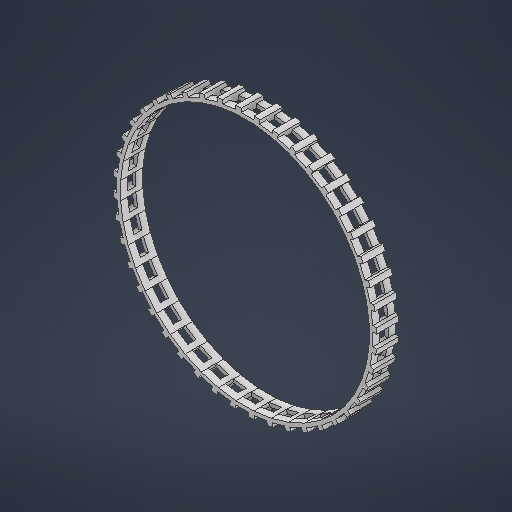
# Autodesk Inventor part: good_track
Saved by Autodesk Inventor 2026.2 (Build 302298010, 298A)
## iProperties
Created: 2026-07-08
Part Number: good_track
Material: Generic
Document SubType Name: Modeling
Designer: vicke
Density: 1 g/cm^3
Appearance: Default
Author: vicke
Autodesk Inventor part; units mm, degrees
ref_plane "YZ Plane" through (0, 0, 0) normal (1, 0, 0) x (0, 1, 0)
ref_plane "XZ Plane" through (0, 0, 0) normal (0, 1, 0) x (-1, 0, 0)
ref_plane "XY Plane" through (0, 0, 0) normal (0, 0, 1) x (1, 0, 0)
sketch "Sketch1" plane through (0, 0, 0) normal (0, 0, 1) x (1, 0, 0)
  line L0 (-5, 67) -> (5, 67)
  line L1 (0, 67) -> (-5, 67)
  line L2 (-5, 67) -> (-5, 71)
  line L3 (0, 67) -> (5, 67)
  line L4 (-5, 71) -> (-2, 71)
  line L5 (-2, 71) -> (-2, 67)
  line L6 (-2, 67) -> (-5, 67)
  line L7 (-5, 67) -> (-5, 71)
  line L8 (5, 67) -> (-2, 67)
  line L9 (-2, 67) -> (-2, 69)
  line L10 (-2, 69) -> (5, 69)
  line L11 (5, 69) -> (5, 67)
  line L12 (-14.4842, 65.6065) -> (-4.586, 67.0296)
  line L13 (-9.5351, 66.318) -> (-14.4842, 65.6065)
  line L14 (-9.5351, 66.318) -> (-4.586, 67.0296)
  line L15 (-11.5147, 66.0334) -> (-14.4842, 65.6065)
  line L16 (-4.586, 67.0296) -> (-11.5147, 66.0334)
  line L17 (-11.5147, 66.0334) -> (-11.7994, 68.013)
  line L18 (-11.7994, 68.013) -> (-4.8706, 69.0093)
  line L19 (-4.8706, 69.0093) -> (-4.586, 67.0296)
  line L20 (-14.4842, 65.6065) -> (-15.0535, 69.5657)
  line L21 (-15.0535, 69.5657) -> (-12.084, 69.9927)
  line L22 (-12.084, 69.9927) -> (-11.5147, 66.0334)
  line L23 (-14.4842, 65.6065) -> (-15.0535, 69.5657)
  line L24 (-23.6735, 62.8774) -> (-14.0786, 65.6947)
  line L25 (-18.8761, 64.286) -> (-23.6735, 62.8774)
  line L26 (-18.8761, 64.286) -> (-14.0786, 65.6947)
  line L27 (-20.7951, 63.7226) -> (-23.6735, 62.8774)
  line L28 (-14.0786, 65.6947) -> (-20.7951, 63.7226)
  line L29 (-20.7951, 63.7226) -> (-21.3585, 65.6416)
  line L30 (-21.3585, 65.6416) -> (-14.6421, 67.6137)
  line L31 (-14.6421, 67.6137) -> (-14.0786, 65.6947)
  line L32 (-23.6735, 62.8774) -> (-24.8005, 66.7153)
  line L33 (-24.8005, 66.7153) -> (-21.922, 67.5605)
  line L34 (-21.922, 67.5605) -> (-20.7951, 63.7226)
  line L35 (-23.6735, 62.8774) -> (-24.8005, 66.7153)
  line L36 (-32.381, 58.8683) -> (-23.2846, 63.0224)
  line L37 (-27.8328, 60.9453) -> (-32.381, 58.8683)
  line L38 (-27.8328, 60.9453) -> (-23.2846, 63.0224)
  line L39 (-29.6521, 60.1145) -> (-32.381, 58.8683)
  line L40 (-23.2846, 63.0224) -> (-29.6521, 60.1145)
  line L41 (-29.6521, 60.1145) -> (-30.4829, 61.9338)
  line L42 (-30.4829, 61.9338) -> (-24.1155, 64.8417)
  line L43 (-24.1155, 64.8417) -> (-23.2846, 63.0224)
  line L44 (-32.381, 58.8683) -> (-34.0426, 62.5068)
  line L45 (-34.0426, 62.5068) -> (-31.3137, 63.753)
  line L46 (-31.3137, 63.753) -> (-29.6521, 60.1145)
  line L47 (-32.381, 58.8683) -> (-34.0426, 62.5068)
  line L48 (-40.4292, 53.6608) -> (-32.0167, 59.0672)
  line L49 (-36.2229, 56.364) -> (-40.4292, 53.6608)
  line L50 (-36.2229, 56.364) -> (-32.0167, 59.0672)
  line L51 (-37.9054, 55.2827) -> (-40.4292, 53.6608)
  line L52 (-32.0167, 59.0672) -> (-37.9054, 55.2827)
  line L53 (-37.9054, 55.2827) -> (-38.9867, 56.9652)
  line L54 (-38.9867, 56.9652) -> (-33.0979, 60.7497)
  line L55 (-33.0979, 60.7497) -> (-32.0167, 59.0672)
  line L56 (-40.4292, 53.6608) -> (-42.5918, 57.0258)
  line L57 (-42.5918, 57.0258) -> (-40.068, 58.6477)
  line L58 (-40.068, 58.6477) -> (-37.9054, 55.2827)
  line L59 (-40.4292, 53.6608) -> (-42.5918, 57.0258)
  line L60 (-47.6544, 47.3609) -> (-40.0969, 53.9095)
  line L61 (-43.8757, 50.6352) -> (-47.6544, 47.3609)
  line L62 (-43.8757, 50.6352) -> (-40.0969, 53.9095)
  line L63 (-45.3872, 49.3255) -> (-47.6544, 47.3609)
  line L64 (-40.0969, 53.9095) -> (-45.3872, 49.3255)
  line L65 (-45.3872, 49.3255) -> (-46.6969, 50.837)
  line L66 (-46.6969, 50.837) -> (-41.4066, 55.421)
  line L67 (-41.4066, 55.421) -> (-40.0969, 53.9095)
  line L68 (-47.6544, 47.3609) -> (-50.2739, 50.3839)
  line L69 (-50.2739, 50.3839) -> (-48.0066, 52.3485)
  line L70 (-48.0066, 52.3485) -> (-45.3872, 49.3255)
  line L71 (-47.6544, 47.3609) -> (-50.2739, 50.3839)
  line L72 (-53.9095, 40.0969) -> (-47.3609, 47.6544)
  line L73 (-50.6352, 43.8757) -> (-53.9095, 40.0969)
  line L74 (-50.6352, 43.8757) -> (-47.3609, 47.6544)
  line L75 (-51.9449, 42.3642) -> (-53.9095, 40.0969)
  line L76 (-47.3609, 47.6544) -> (-51.9449, 42.3642)
  line L77 (-51.9449, 42.3642) -> (-53.4564, 43.6739)
  line L78 (-53.4564, 43.6739) -> (-48.8724, 48.9641)
  line L79 (-48.8724, 48.9641) -> (-47.3609, 47.6544)
  line L80 (-53.9095, 40.0969) -> (-56.9325, 42.7164)
  line L81 (-56.9325, 42.7164) -> (-54.9679, 44.9836)
  line L82 (-54.9679, 44.9836) -> (-51.9449, 42.3642)
  line L83 (-53.9095, 40.0969) -> (-56.9325, 42.7164)
  line L84 (-59.0672, 32.0167) -> (-53.6608, 40.4292)
  line L85 (-56.364, 36.2229) -> (-59.0672, 32.0167)
  line L86 (-56.364, 36.2229) -> (-53.6608, 40.4292)
  line L87 (-57.4453, 34.5404) -> (-59.0672, 32.0167)
  line L88 (-53.6608, 40.4292) -> (-57.4453, 34.5404)
  line L89 (-57.4453, 34.5404) -> (-59.1278, 35.6217)
  line L90 (-59.1278, 35.6217) -> (-55.3433, 41.5105)
  line L91 (-55.3433, 41.5105) -> (-53.6608, 40.4292)
  line L92 (-59.0672, 32.0167) -> (-62.4322, 34.1792)
  line L93 (-62.4322, 34.1792) -> (-60.8103, 36.703)
  line L94 (-60.8103, 36.703) -> (-57.4453, 34.5404)
  line L95 (-59.0672, 32.0167) -> (-62.4322, 34.1792)
  line L96 (-63.0224, 23.2846) -> (-58.8683, 32.381)
  line L97 (-60.9453, 27.8328) -> (-63.0224, 23.2846)
  line L98 (-60.9453, 27.8328) -> (-58.8683, 32.381)
  line L99 (-61.7762, 26.0135) -> (-63.0224, 23.2846)
  line L100 (-58.8683, 32.381) -> (-61.7762, 26.0135)
  line L101 (-61.7762, 26.0135) -> (-63.5954, 26.8444)
  line L102 (-63.5954, 26.8444) -> (-60.6875, 33.2118)
  line L103 (-60.6875, 33.2118) -> (-58.8683, 32.381)
  line L104 (-63.0224, 23.2846) -> (-66.6609, 24.9463)
  line L105 (-66.6609, 24.9463) -> (-65.4147, 27.6752)
  line L106 (-65.4147, 27.6752) -> (-61.7762, 26.0135)
  line L107 (-63.0224, 23.2846) -> (-66.6609, 24.9463)
  line L108 (-65.6947, 14.0786) -> (-62.8774, 23.6735)
  line L109 (-64.286, 18.8761) -> (-65.6947, 14.0786)
  line L110 (-64.286, 18.8761) -> (-62.8774, 23.6735)
  line L111 (-64.8495, 16.9571) -> (-65.6947, 14.0786)
  line L112 (-62.8774, 23.6735) -> (-64.8495, 16.9571)
  line L113 (-64.8495, 16.9571) -> (-66.7685, 17.5206)
  line L114 (-66.7685, 17.5206) -> (-64.7964, 24.237)
  line L115 (-64.7964, 24.237) -> (-62.8774, 23.6735)
  line L116 (-65.6947, 14.0786) -> (-69.5327, 15.2055)
  line L117 (-69.5327, 15.2055) -> (-68.6875, 18.084)
  line L118 (-68.6875, 18.084) -> (-64.8495, 16.9571)
  line L119 (-65.6947, 14.0786) -> (-69.5327, 15.2055)
  line L120 (-67.0296, 4.586) -> (-65.6065, 14.4842)
  line L121 (-66.318, 9.5351) -> (-67.0296, 4.586)
  line L122 (-66.318, 9.5351) -> (-65.6065, 14.4842)
  line L123 (-66.6027, 7.5555) -> (-67.0296, 4.586)
  line L124 (-65.6065, 14.4842) -> (-66.6027, 7.5555)
  line L125 (-66.6027, 7.5555) -> (-68.5823, 7.8401)
  line L126 (-68.5823, 7.8401) -> (-67.5861, 14.7688)
  line L127 (-67.5861, 14.7688) -> (-65.6065, 14.4842)
  line L128 (-67.0296, 4.586) -> (-70.9889, 5.1552)
  line L129 (-70.9889, 5.1552) -> (-70.562, 8.1247)
  line L130 (-70.562, 8.1247) -> (-66.6027, 7.5555)
  line L131 (-67.0296, 4.586) -> (-70.9889, 5.1552)
  line L132 (-67, -5) -> (-67, 5)
  line L133 (-67, 0) -> (-67, -5)
  line L134 (-67, 0) -> (-67, 5)
  line L135 (-67, -2) -> (-67, -5)
  line L136 (-67, 5) -> (-67, -2)
  line L137 (-67, -2) -> (-69, -2)
  line L138 (-69, -2) -> (-69, 5)
  line L139 (-69, 5) -> (-67, 5)
  line L140 (-67, -5) -> (-71, -5)
  line L141 (-71, -5) -> (-71, -2)
  line L142 (-71, -2) -> (-67, -2)
  line L143 (-67, -5) -> (-71, -5)
  line L144 (-65.6065, -14.4842) -> (-67.0296, -4.586)
  line L145 (-66.318, -9.5351) -> (-65.6065, -14.4842)
  line L146 (-66.318, -9.5351) -> (-67.0296, -4.586)
  line L147 (-66.0334, -11.5147) -> (-65.6065, -14.4842)
  line L148 (-67.0296, -4.586) -> (-66.0334, -11.5147)
  line L149 (-66.0334, -11.5147) -> (-68.013, -11.7994)
  line L150 (-68.013, -11.7994) -> (-69.0093, -4.8706)
  line L151 (-69.0093, -4.8706) -> (-67.0296, -4.586)
  line L152 (-65.6065, -14.4842) -> (-69.5657, -15.0535)
  line L153 (-69.5657, -15.0535) -> (-69.9927, -12.084)
  line L154 (-69.9927, -12.084) -> (-66.0334, -11.5147)
  line L155 (-65.6065, -14.4842) -> (-69.5657, -15.0535)
  line L156 (-62.8774, -23.6735) -> (-65.6947, -14.0786)
  line L157 (-64.286, -18.8761) -> (-62.8774, -23.6735)
  line L158 (-64.286, -18.8761) -> (-65.6947, -14.0786)
  line L159 (-63.7226, -20.7951) -> (-62.8774, -23.6735)
  line L160 (-65.6947, -14.0786) -> (-63.7226, -20.7951)
  line L161 (-63.7226, -20.7951) -> (-65.6416, -21.3585)
  line L162 (-65.6416, -21.3585) -> (-67.6137, -14.6421)
  line L163 (-67.6137, -14.6421) -> (-65.6947, -14.0786)
  line L164 (-62.8774, -23.6735) -> (-66.7153, -24.8005)
  line L165 (-66.7153, -24.8005) -> (-67.5605, -21.922)
  line L166 (-67.5605, -21.922) -> (-63.7226, -20.7951)
  line L167 (-62.8774, -23.6735) -> (-66.7153, -24.8005)
  line L168 (-58.8683, -32.381) -> (-63.0224, -23.2846)
  line L169 (-60.9453, -27.8328) -> (-58.8683, -32.381)
  line L170 (-60.9453, -27.8328) -> (-63.0224, -23.2846)
  line L171 (-60.1145, -29.6521) -> (-58.8683, -32.381)
  line L172 (-63.0224, -23.2846) -> (-60.1145, -29.6521)
  line L173 (-60.1145, -29.6521) -> (-61.9338, -30.4829)
  line L174 (-61.9338, -30.4829) -> (-64.8417, -24.1155)
  line L175 (-64.8417, -24.1155) -> (-63.0224, -23.2846)
  line L176 (-58.8683, -32.381) -> (-62.5068, -34.0426)
  line L177 (-62.5068, -34.0426) -> (-63.753, -31.3137)
  line L178 (-63.753, -31.3137) -> (-60.1145, -29.6521)
  line L179 (-58.8683, -32.381) -> (-62.5068, -34.0426)
  line L180 (-53.6608, -40.4292) -> (-59.0672, -32.0167)
  line L181 (-56.364, -36.2229) -> (-53.6608, -40.4292)
  line L182 (-56.364, -36.2229) -> (-59.0672, -32.0167)
  line L183 (-55.2827, -37.9054) -> (-53.6608, -40.4292)
  line L184 (-59.0672, -32.0167) -> (-55.2827, -37.9054)
  line L185 (-55.2827, -37.9054) -> (-56.9652, -38.9867)
  line L186 (-56.9652, -38.9867) -> (-60.7497, -33.0979)
  line L187 (-60.7497, -33.0979) -> (-59.0672, -32.0167)
  line L188 (-53.6608, -40.4292) -> (-57.0258, -42.5918)
  line L189 (-57.0258, -42.5918) -> (-58.6477, -40.068)
  line L190 (-58.6477, -40.068) -> (-55.2827, -37.9054)
  line L191 (-53.6608, -40.4292) -> (-57.0258, -42.5918)
  line L192 (-47.3609, -47.6544) -> (-53.9095, -40.0969)
  line L193 (-50.6352, -43.8757) -> (-47.3609, -47.6544)
  line L194 (-50.6352, -43.8757) -> (-53.9095, -40.0969)
  line L195 (-49.3255, -45.3872) -> (-47.3609, -47.6544)
  line L196 (-53.9095, -40.0969) -> (-49.3255, -45.3872)
  line L197 (-49.3255, -45.3872) -> (-50.837, -46.6969)
  line L198 (-50.837, -46.6969) -> (-55.421, -41.4066)
  line L199 (-55.421, -41.4066) -> (-53.9095, -40.0969)
  line L200 (-47.3609, -47.6544) -> (-50.3839, -50.2739)
  line L201 (-50.3839, -50.2739) -> (-52.3485, -48.0066)
  line L202 (-52.3485, -48.0066) -> (-49.3255, -45.3872)
  line L203 (-47.3609, -47.6544) -> (-50.3839, -50.2739)
  line L204 (-40.0969, -53.9095) -> (-47.6544, -47.3609)
  line L205 (-43.8757, -50.6352) -> (-40.0969, -53.9095)
  line L206 (-43.8757, -50.6352) -> (-47.6544, -47.3609)
  line L207 (-42.3642, -51.9449) -> (-40.0969, -53.9095)
  line L208 (-47.6544, -47.3609) -> (-42.3642, -51.9449)
  line L209 (-42.3642, -51.9449) -> (-43.6739, -53.4564)
  line L210 (-43.6739, -53.4564) -> (-48.9641, -48.8724)
  line L211 (-48.9641, -48.8724) -> (-47.6544, -47.3609)
  line L212 (-40.0969, -53.9095) -> (-42.7164, -56.9325)
  line L213 (-42.7164, -56.9325) -> (-44.9836, -54.9679)
  line L214 (-44.9836, -54.9679) -> (-42.3642, -51.9449)
  line L215 (-40.0969, -53.9095) -> (-42.7164, -56.9325)
  line L216 (-32.0167, -59.0672) -> (-40.4292, -53.6608)
  line L217 (-36.2229, -56.364) -> (-32.0167, -59.0672)
  line L218 (-36.2229, -56.364) -> (-40.4292, -53.6608)
  line L219 (-34.5404, -57.4453) -> (-32.0167, -59.0672)
  line L220 (-40.4292, -53.6608) -> (-34.5404, -57.4453)
  line L221 (-34.5404, -57.4453) -> (-35.6217, -59.1278)
  line L222 (-35.6217, -59.1278) -> (-41.5105, -55.3433)
  line L223 (-41.5105, -55.3433) -> (-40.4292, -53.6608)
  line L224 (-32.0167, -59.0672) -> (-34.1792, -62.4322)
  line L225 (-34.1792, -62.4322) -> (-36.703, -60.8103)
  line L226 (-36.703, -60.8103) -> (-34.5404, -57.4453)
  line L227 (-32.0167, -59.0672) -> (-34.1792, -62.4322)
  line L228 (-23.2846, -63.0224) -> (-32.381, -58.8683)
  line L229 (-27.8328, -60.9453) -> (-23.2846, -63.0224)
  line L230 (-27.8328, -60.9453) -> (-32.381, -58.8683)
  line L231 (-26.0135, -61.7762) -> (-23.2846, -63.0224)
  line L232 (-32.381, -58.8683) -> (-26.0135, -61.7762)
  line L233 (-26.0135, -61.7762) -> (-26.8444, -63.5954)
  line L234 (-26.8444, -63.5954) -> (-33.2118, -60.6875)
  line L235 (-33.2118, -60.6875) -> (-32.381, -58.8683)
  line L236 (-23.2846, -63.0224) -> (-24.9463, -66.6609)
  line L237 (-24.9463, -66.6609) -> (-27.6752, -65.4147)
  line L238 (-27.6752, -65.4147) -> (-26.0135, -61.7762)
  line L239 (-23.2846, -63.0224) -> (-24.9463, -66.6609)
  line L240 (-14.0786, -65.6947) -> (-23.6735, -62.8774)
  line L241 (-18.8761, -64.286) -> (-14.0786, -65.6947)
  line L242 (-18.8761, -64.286) -> (-23.6735, -62.8774)
  line L243 (-16.9571, -64.8495) -> (-14.0786, -65.6947)
  line L244 (-23.6735, -62.8774) -> (-16.9571, -64.8495)
  line L245 (-16.9571, -64.8495) -> (-17.5206, -66.7685)
  line L246 (-17.5206, -66.7685) -> (-24.237, -64.7964)
  line L247 (-24.237, -64.7964) -> (-23.6735, -62.8774)
  line L248 (-14.0786, -65.6947) -> (-15.2055, -69.5327)
  line L249 (-15.2055, -69.5327) -> (-18.084, -68.6875)
  line L250 (-18.084, -68.6875) -> (-16.9571, -64.8495)
  line L251 (-14.0786, -65.6947) -> (-15.2055, -69.5327)
  line L252 (-4.586, -67.0296) -> (-14.4842, -65.6065)
  line L253 (-9.5351, -66.318) -> (-4.586, -67.0296)
  line L254 (-9.5351, -66.318) -> (-14.4842, -65.6065)
  line L255 (-7.5555, -66.6027) -> (-4.586, -67.0296)
  line L256 (-14.4842, -65.6065) -> (-7.5555, -66.6027)
  line L257 (-7.5555, -66.6027) -> (-7.8401, -68.5823)
  line L258 (-7.8401, -68.5823) -> (-14.7688, -67.5861)
  line L259 (-14.7688, -67.5861) -> (-14.4842, -65.6065)
  line L260 (-4.586, -67.0296) -> (-5.1552, -70.9889)
  line L261 (-5.1552, -70.9889) -> (-8.1247, -70.562)
  line L262 (-8.1247, -70.562) -> (-7.5555, -66.6027)
  line L263 (-4.586, -67.0296) -> (-5.1552, -70.9889)
  line L264 (5, -67) -> (-5, -67)
  line L265 (0, -67) -> (5, -67)
  line L266 (0, -67) -> (-5, -67)
  line L267 (2, -67) -> (5, -67)
  line L268 (-5, -67) -> (2, -67)
  line L269 (2, -67) -> (2, -69)
  line L270 (2, -69) -> (-5, -69)
  line L271 (-5, -69) -> (-5, -67)
  line L272 (5, -67) -> (5, -71)
  line L273 (5, -71) -> (2, -71)
  line L274 (2, -71) -> (2, -67)
  line L275 (5, -67) -> (5, -71)
  line L276 (14.4842, -65.6065) -> (4.586, -67.0296)
  line L277 (9.5351, -66.318) -> (14.4842, -65.6065)
  line L278 (9.5351, -66.318) -> (4.586, -67.0296)
  line L279 (11.5147, -66.0334) -> (14.4842, -65.6065)
  line L280 (4.586, -67.0296) -> (11.5147, -66.0334)
  line L281 (11.5147, -66.0334) -> (11.7994, -68.013)
  line L282 (11.7994, -68.013) -> (4.8706, -69.0093)
  line L283 (4.8706, -69.0093) -> (4.586, -67.0296)
  line L284 (14.4842, -65.6065) -> (15.0535, -69.5657)
  line L285 (15.0535, -69.5657) -> (12.084, -69.9927)
  line L286 (12.084, -69.9927) -> (11.5147, -66.0334)
  line L287 (14.4842, -65.6065) -> (15.0535, -69.5657)
  line L288 (23.6735, -62.8774) -> (14.0786, -65.6947)
  line L289 (18.8761, -64.286) -> (23.6735, -62.8774)
  line L290 (18.8761, -64.286) -> (14.0786, -65.6947)
  line L291 (20.7951, -63.7226) -> (23.6735, -62.8774)
  line L292 (14.0786, -65.6947) -> (20.7951, -63.7226)
  line L293 (20.7951, -63.7226) -> (21.3585, -65.6416)
  line L294 (21.3585, -65.6416) -> (14.6421, -67.6137)
  line L295 (14.6421, -67.6137) -> (14.0786, -65.6947)
  line L296 (23.6735, -62.8774) -> (24.8005, -66.7153)
  line L297 (24.8005, -66.7153) -> (21.922, -67.5605)
  line L298 (21.922, -67.5605) -> (20.7951, -63.7226)
  line L299 (23.6735, -62.8774) -> (24.8005, -66.7153)
  line L300 (32.381, -58.8683) -> (23.2846, -63.0224)
  line L301 (27.8328, -60.9453) -> (32.381, -58.8683)
  line L302 (27.8328, -60.9453) -> (23.2846, -63.0224)
  line L303 (29.6521, -60.1145) -> (32.381, -58.8683)
  line L304 (23.2846, -63.0224) -> (29.6521, -60.1145)
  line L305 (29.6521, -60.1145) -> (30.4829, -61.9338)
  line L306 (30.4829, -61.9338) -> (24.1155, -64.8417)
  line L307 (24.1155, -64.8417) -> (23.2846, -63.0224)
  line L308 (32.381, -58.8683) -> (34.0426, -62.5068)
  line L309 (34.0426, -62.5068) -> (31.3137, -63.753)
  line L310 (31.3137, -63.753) -> (29.6521, -60.1145)
  line L311 (32.381, -58.8683) -> (34.0426, -62.5068)
  line L312 (40.4292, -53.6608) -> (32.0167, -59.0672)
  line L313 (36.2229, -56.364) -> (40.4292, -53.6608)
  line L314 (36.2229, -56.364) -> (32.0167, -59.0672)
  line L315 (37.9054, -55.2827) -> (40.4292, -53.6608)
  line L316 (32.0167, -59.0672) -> (37.9054, -55.2827)
  line L317 (37.9054, -55.2827) -> (38.9867, -56.9652)
  line L318 (38.9867, -56.9652) -> (33.0979, -60.7497)
  line L319 (33.0979, -60.7497) -> (32.0167, -59.0672)
  line L320 (40.4292, -53.6608) -> (42.5918, -57.0258)
  line L321 (42.5918, -57.0258) -> (40.068, -58.6477)
  line L322 (40.068, -58.6477) -> (37.9054, -55.2827)
  line L323 (40.4292, -53.6608) -> (42.5918, -57.0258)
  line L324 (47.6544, -47.3609) -> (40.0969, -53.9095)
  line L325 (43.8757, -50.6352) -> (47.6544, -47.3609)
  line L326 (43.8757, -50.6352) -> (40.0969, -53.9095)
  line L327 (45.3872, -49.3255) -> (47.6544, -47.3609)
  line L328 (40.0969, -53.9095) -> (45.3872, -49.3255)
  line L329 (45.3872, -49.3255) -> (46.6969, -50.837)
  line L330 (46.6969, -50.837) -> (41.4066, -55.421)
  line L331 (41.4066, -55.421) -> (40.0969, -53.9095)
  line L332 (47.6544, -47.3609) -> (50.2739, -50.3839)
  line L333 (50.2739, -50.3839) -> (48.0066, -52.3485)
  line L334 (48.0066, -52.3485) -> (45.3872, -49.3255)
  line L335 (47.6544, -47.3609) -> (50.2739, -50.3839)
  line L336 (53.9095, -40.0969) -> (47.3609, -47.6544)
  line L337 (50.6352, -43.8757) -> (53.9095, -40.0969)
  line L338 (50.6352, -43.8757) -> (47.3609, -47.6544)
  line L339 (51.9449, -42.3642) -> (53.9095, -40.0969)
  line L340 (47.3609, -47.6544) -> (51.9449, -42.3642)
  line L341 (51.9449, -42.3642) -> (53.4564, -43.6739)
  line L342 (53.4564, -43.6739) -> (48.8724, -48.9641)
  line L343 (48.8724, -48.9641) -> (47.3609, -47.6544)
  line L344 (53.9095, -40.0969) -> (56.9325, -42.7164)
  line L345 (56.9325, -42.7164) -> (54.9679, -44.9836)
  line L346 (54.9679, -44.9836) -> (51.9449, -42.3642)
  line L347 (53.9095, -40.0969) -> (56.9325, -42.7164)
  line L348 (59.0672, -32.0167) -> (53.6608, -40.4292)
  line L349 (56.364, -36.2229) -> (59.0672, -32.0167)
  line L350 (56.364, -36.2229) -> (53.6608, -40.4292)
  line L351 (57.4453, -34.5404) -> (59.0672, -32.0167)
  line L352 (53.6608, -40.4292) -> (57.4453, -34.5404)
  line L353 (57.4453, -34.5404) -> (59.1278, -35.6217)
  line L354 (59.1278, -35.6217) -> (55.3433, -41.5105)
  line L355 (55.3433, -41.5105) -> (53.6608, -40.4292)
  line L356 (59.0672, -32.0167) -> (62.4322, -34.1792)
  line L357 (62.4322, -34.1792) -> (60.8103, -36.703)
  line L358 (60.8103, -36.703) -> (57.4453, -34.5404)
  line L359 (59.0672, -32.0167) -> (62.4322, -34.1792)
  line L360 (63.0224, -23.2846) -> (58.8683, -32.381)
  line L361 (60.9453, -27.8328) -> (63.0224, -23.2846)
  line L362 (60.9453, -27.8328) -> (58.8683, -32.381)
  line L363 (61.7762, -26.0135) -> (63.0224, -23.2846)
  line L364 (58.8683, -32.381) -> (61.7762, -26.0135)
  line L365 (61.7762, -26.0135) -> (63.5954, -26.8444)
  line L366 (63.5954, -26.8444) -> (60.6875, -33.2118)
  line L367 (60.6875, -33.2118) -> (58.8683, -32.381)
  line L368 (63.0224, -23.2846) -> (66.6609, -24.9463)
  line L369 (66.6609, -24.9463) -> (65.4147, -27.6752)
  line L370 (65.4147, -27.6752) -> (61.7762, -26.0135)
  line L371 (63.0224, -23.2846) -> (66.6609, -24.9463)
  line L372 (65.6947, -14.0786) -> (62.8774, -23.6735)
  line L373 (64.286, -18.8761) -> (65.6947, -14.0786)
  line L374 (64.286, -18.8761) -> (62.8774, -23.6735)
  line L375 (64.8495, -16.9571) -> (65.6947, -14.0786)
  line L376 (62.8774, -23.6735) -> (64.8495, -16.9571)
  line L377 (64.8495, -16.9571) -> (66.7685, -17.5206)
  line L378 (66.7685, -17.5206) -> (64.7964, -24.237)
  line L379 (64.7964, -24.237) -> (62.8774, -23.6735)
  line L380 (65.6947, -14.0786) -> (69.5327, -15.2055)
  line L381 (69.5327, -15.2055) -> (68.6875, -18.084)
  line L382 (68.6875, -18.084) -> (64.8495, -16.9571)
  line L383 (65.6947, -14.0786) -> (69.5327, -15.2055)
  line L384 (67.0296, -4.586) -> (65.6065, -14.4842)
  line L385 (66.318, -9.5351) -> (67.0296, -4.586)
  line L386 (66.318, -9.5351) -> (65.6065, -14.4842)
  line L387 (66.6027, -7.5555) -> (67.0296, -4.586)
  line L388 (65.6065, -14.4842) -> (66.6027, -7.5555)
  line L389 (66.6027, -7.5555) -> (68.5823, -7.8401)
  line L390 (68.5823, -7.8401) -> (67.5861, -14.7688)
  line L391 (67.5861, -14.7688) -> (65.6065, -14.4842)
  line L392 (67.0296, -4.586) -> (70.9889, -5.1552)
  line L393 (70.9889, -5.1552) -> (70.562, -8.1247)
  line L394 (70.562, -8.1247) -> (66.6027, -7.5555)
  line L395 (67.0296, -4.586) -> (70.9889, -5.1552)
  line L396 (67, 5) -> (67, -5)
  line L397 (67, 0) -> (67, 5)
  line L398 (67, 0) -> (67, -5)
  line L399 (67, 2) -> (67, 5)
  line L400 (67, -5) -> (67, 2)
  line L401 (67, 2) -> (69, 2)
  line L402 (69, 2) -> (69, -5)
  line L403 (69, -5) -> (67, -5)
  line L404 (67, 5) -> (71, 5)
  line L405 (71, 5) -> (71, 2)
  line L406 (71, 2) -> (67, 2)
  line L407 (67, 5) -> (71, 5)
  line L408 (65.6065, 14.4842) -> (67.0296, 4.586)
  line L409 (66.318, 9.5351) -> (65.6065, 14.4842)
  line L410 (66.318, 9.5351) -> (67.0296, 4.586)
  line L411 (66.0334, 11.5147) -> (65.6065, 14.4842)
  line L412 (67.0296, 4.586) -> (66.0334, 11.5147)
  line L413 (66.0334, 11.5147) -> (68.013, 11.7994)
  line L414 (68.013, 11.7994) -> (69.0093, 4.8706)
  line L415 (69.0093, 4.8706) -> (67.0296, 4.586)
  line L416 (65.6065, 14.4842) -> (69.5657, 15.0535)
  line L417 (69.5657, 15.0535) -> (69.9927, 12.084)
  line L418 (69.9927, 12.084) -> (66.0334, 11.5147)
  line L419 (65.6065, 14.4842) -> (69.5657, 15.0535)
  line L420 (62.8774, 23.6735) -> (65.6947, 14.0786)
  line L421 (64.286, 18.8761) -> (62.8774, 23.6735)
  line L422 (64.286, 18.8761) -> (65.6947, 14.0786)
  line L423 (63.7226, 20.7951) -> (62.8774, 23.6735)
  line L424 (65.6947, 14.0786) -> (63.7226, 20.7951)
  line L425 (63.7226, 20.7951) -> (65.6416, 21.3585)
  line L426 (65.6416, 21.3585) -> (67.6137, 14.6421)
  line L427 (67.6137, 14.6421) -> (65.6947, 14.0786)
  line L428 (62.8774, 23.6735) -> (66.7153, 24.8005)
  line L429 (66.7153, 24.8005) -> (67.5605, 21.922)
  line L430 (67.5605, 21.922) -> (63.7226, 20.7951)
  line L431 (62.8774, 23.6735) -> (66.7153, 24.8005)
  line L432 (58.8683, 32.381) -> (63.0224, 23.2846)
  line L433 (60.9453, 27.8328) -> (58.8683, 32.381)
  line L434 (60.9453, 27.8328) -> (63.0224, 23.2846)
  line L435 (60.1145, 29.6521) -> (58.8683, 32.381)
  line L436 (63.0224, 23.2846) -> (60.1145, 29.6521)
  line L437 (60.1145, 29.6521) -> (61.9338, 30.4829)
  line L438 (61.9338, 30.4829) -> (64.8417, 24.1155)
  line L439 (64.8417, 24.1155) -> (63.0224, 23.2846)
  line L440 (58.8683, 32.381) -> (62.5068, 34.0426)
  line L441 (62.5068, 34.0426) -> (63.753, 31.3137)
  line L442 (63.753, 31.3137) -> (60.1145, 29.6521)
  line L443 (58.8683, 32.381) -> (62.5068, 34.0426)
  line L444 (53.6608, 40.4292) -> (59.0672, 32.0167)
  line L445 (56.364, 36.2229) -> (53.6608, 40.4292)
  line L446 (56.364, 36.2229) -> (59.0672, 32.0167)
  line L447 (55.2827, 37.9054) -> (53.6608, 40.4292)
  line L448 (59.0672, 32.0167) -> (55.2827, 37.9054)
  line L449 (55.2827, 37.9054) -> (56.9652, 38.9867)
  line L450 (56.9652, 38.9867) -> (60.7497, 33.0979)
  line L451 (60.7497, 33.0979) -> (59.0672, 32.0167)
  line L452 (53.6608, 40.4292) -> (57.0258, 42.5918)
  line L453 (57.0258, 42.5918) -> (58.6477, 40.068)
  line L454 (58.6477, 40.068) -> (55.2827, 37.9054)
  line L455 (53.6608, 40.4292) -> (57.0258, 42.5918)
  line L456 (47.3609, 47.6544) -> (53.9095, 40.0969)
  line L457 (50.6352, 43.8757) -> (47.3609, 47.6544)
  line L458 (50.6352, 43.8757) -> (53.9095, 40.0969)
  line L459 (49.3255, 45.3872) -> (47.3609, 47.6544)
  line L460 (53.9095, 40.0969) -> (49.3255, 45.3872)
  line L461 (49.3255, 45.3872) -> (50.837, 46.6969)
  line L462 (50.837, 46.6969) -> (55.421, 41.4066)
  line L463 (55.421, 41.4066) -> (53.9095, 40.0969)
  line L464 (47.3609, 47.6544) -> (50.3839, 50.2739)
  line L465 (50.3839, 50.2739) -> (52.3485, 48.0066)
  line L466 (52.3485, 48.0066) -> (49.3255, 45.3872)
  line L467 (47.3609, 47.6544) -> (50.3839, 50.2739)
  line L468 (40.0969, 53.9095) -> (47.6544, 47.3609)
  line L469 (43.8757, 50.6352) -> (40.0969, 53.9095)
  line L470 (43.8757, 50.6352) -> (47.6544, 47.3609)
  line L471 (42.3642, 51.9449) -> (40.0969, 53.9095)
  line L472 (47.6544, 47.3609) -> (42.3642, 51.9449)
  line L473 (42.3642, 51.9449) -> (43.6739, 53.4564)
  line L474 (43.6739, 53.4564) -> (48.9641, 48.8724)
  line L475 (48.9641, 48.8724) -> (47.6544, 47.3609)
  line L476 (40.0969, 53.9095) -> (42.7164, 56.9325)
  line L477 (42.7164, 56.9325) -> (44.9836, 54.9679)
  line L478 (44.9836, 54.9679) -> (42.3642, 51.9449)
  line L479 (40.0969, 53.9095) -> (42.7164, 56.9325)
  line L480 (32.0167, 59.0672) -> (40.4292, 53.6608)
  line L481 (36.2229, 56.364) -> (32.0167, 59.0672)
  line L482 (36.2229, 56.364) -> (40.4292, 53.6608)
  line L483 (34.5404, 57.4453) -> (32.0167, 59.0672)
  line L484 (40.4292, 53.6608) -> (34.5404, 57.4453)
  line L485 (34.5404, 57.4453) -> (35.6217, 59.1278)
  line L486 (35.6217, 59.1278) -> (41.5105, 55.3433)
  line L487 (41.5105, 55.3433) -> (40.4292, 53.6608)
  line L488 (32.0167, 59.0672) -> (34.1792, 62.4322)
  line L489 (34.1792, 62.4322) -> (36.703, 60.8103)
  line L490 (36.703, 60.8103) -> (34.5404, 57.4453)
  line L491 (32.0167, 59.0672) -> (34.1792, 62.4322)
  line L492 (23.2846, 63.0224) -> (32.381, 58.8683)
  line L493 (27.8328, 60.9453) -> (23.2846, 63.0224)
  line L494 (27.8328, 60.9453) -> (32.381, 58.8683)
  line L495 (26.0135, 61.7762) -> (23.2846, 63.0224)
  line L496 (32.381, 58.8683) -> (26.0135, 61.7762)
  line L497 (26.0135, 61.7762) -> (26.8444, 63.5954)
  line L498 (26.8444, 63.5954) -> (33.2118, 60.6875)
  line L499 (33.2118, 60.6875) -> (32.381, 58.8683)
  line L500 (23.2846, 63.0224) -> (24.9463, 66.6609)
  line L501 (24.9463, 66.6609) -> (27.6752, 65.4147)
  line L502 (27.6752, 65.4147) -> (26.0135, 61.7762)
  line L503 (23.2846, 63.0224) -> (24.9463, 66.6609)
  line L504 (14.0786, 65.6947) -> (23.6735, 62.8774)
  line L505 (18.8761, 64.286) -> (14.0786, 65.6947)
  line L506 (18.8761, 64.286) -> (23.6735, 62.8774)
  line L507 (16.9571, 64.8495) -> (14.0786, 65.6947)
  line L508 (23.6735, 62.8774) -> (16.9571, 64.8495)
  line L509 (16.9571, 64.8495) -> (17.5206, 66.7685)
  line L510 (17.5206, 66.7685) -> (24.237, 64.7964)
  line L511 (24.237, 64.7964) -> (23.6735, 62.8774)
  line L512 (14.0786, 65.6947) -> (15.2055, 69.5327)
  line L513 (15.2055, 69.5327) -> (18.084, 68.6875)
  line L514 (18.084, 68.6875) -> (16.9571, 64.8495)
  line L515 (14.0786, 65.6947) -> (15.2055, 69.5327)
  line L516 (4.586, 67.0296) -> (14.4842, 65.6065)
  line L517 (9.5351, 66.318) -> (4.586, 67.0296)
  line L518 (9.5351, 66.318) -> (14.4842, 65.6065)
  line L519 (7.5555, 66.6027) -> (4.586, 67.0296)
  line L520 (14.4842, 65.6065) -> (7.5555, 66.6027)
  line L521 (7.5555, 66.6027) -> (7.8401, 68.5823)
  line L522 (7.8401, 68.5823) -> (14.7688, 67.5861)
  line L523 (14.7688, 67.5861) -> (14.4842, 65.6065)
  line L524 (4.586, 67.0296) -> (5.1552, 70.9889)
  line L525 (5.1552, 70.9889) -> (8.1247, 70.562)
  line L526 (8.1247, 70.562) -> (7.5555, 66.6027)
  line L527 (4.586, 67.0296) -> (5.1552, 70.9889)
  point P0 (0, 0)
  point P1 (14.7675, -67.5769)
  point P2 (24.2344, -64.7874)
  point P3 (33.2079, -60.679)
  point P4 (41.5054, -55.3354)
  point P5 (48.958, -48.8654)
  point P6 (55.414, -41.4005)
  point P7 (60.7418, -33.0929)
  point P8 (64.8332, -24.1116)
  point P9 (67.6047, -14.6394)
  point P10 (8.7848, 72)
  point P11 (6.6842, 70)
  point P12 (65.6361, -14.2783)
  point P13 (62.936, -23.4739)
  point P14 (58.9547, -32.1917)
  point P15 (53.7733, -40.2542)
  point P16 (47.4972, -47.4972)
  point P17 (40.2542, -53.7733)
  point P18 (32.1917, -58.9547)
  point P19 (23.4739, -62.936)
  point P20 (14.2783, -65.6361)
  point P21 (4.7919, -67)
  point P22 (-4.7919, -67)
  point P23 (-14.2783, -65.6361)
  point P24 (-23.4739, -62.936)
  point P25 (-32.1917, -58.9547)
  point P26 (-40.2542, -53.7733)
  point P27 (-47.4972, -47.4972)
  point P28 (-53.7733, -40.2542)
  point P29 (-58.9547, -32.1917)
  point P30 (-62.936, -23.4739)
  point P31 (-65.6361, -14.2783)
  point P32 (-67, -4.7919)
  point P33 (-67, 4.7919)
  point P34 (-65.6361, 14.2783)
  point P35 (-62.936, 23.4739)
  point P36 (-58.9547, 32.1917)
  point P37 (-53.7733, 40.2542)
  point P38 (-47.4972, 47.4972)
  point P39 (-40.2542, 53.7733)
  point P40 (-32.1917, 58.9547)
  point P41 (-23.4739, 62.936)
  point P42 (-14.2783, 65.6361)
  point P43 (-4.7919, 67)
  point P44 (-5, 68.9907)
  point P45 (-14.7675, 67.5769)
  point P46 (-24.2344, 64.7874)
  point P47 (-33.2079, 60.679)
  point P48 (-41.5054, 55.3354)
  point P49 (-48.958, 48.8654)
  point P50 (-55.414, 41.4005)
  point P51 (-60.7418, 33.0929)
  point P52 (-64.8332, 24.1116)
  point P53 (-67.6047, 14.6394)
  point P54 (-69, 4.8693)
  point P55 (-68.9907, -5)
  point P56 (-67.5769, -14.7675)
  point P57 (-64.7874, -24.2344)
  point P58 (-60.679, -33.2079)
  point P59 (-55.3354, -41.5054)
  point P60 (-48.8654, -48.958)
  point P61 (-41.4005, -55.414)
  point P62 (-33.0929, -60.7418)
  point P63 (-24.1116, -64.8332)
  point P64 (-14.6394, -67.6047)
  point P65 (-4.8693, -69)
  point P66 (5, -68.9907)
  point P67 (16.6901, 66.9809)
  point P68 (7.4141, 68.6297)
  point P69 (14.2783, -65.6361)
  point P70 (14.6394, 67.6047)
  point P71 (14.2783, 65.6361)
  point P72 (23.4739, 62.936)
  point P73 (32.1917, 58.9547)
  point P74 (40.2542, 53.7733)
  point P75 (47.4972, 47.4972)
  point P76 (53.7733, 40.2542)
  point P77 (58.9547, 32.1917)
  point P78 (62.936, 23.4739)
  point P79 (65.6361, 14.2783)
  point P80 (67, 4.7919)
  point P81 (67, -4.7919)
  point P82 (69, -4.8693)
  point P83 (68.9907, 5)
  point P84 (67.5769, 14.7675)
  point P85 (64.7874, 24.2344)
  point P86 (60.679, 33.2079)
  point P87 (55.3354, 41.5054)
  point P88 (48.8654, 48.958)
  point P89 (41.4005, 55.414)
  point P90 (33.0929, 60.7418)
  point P91 (24.1116, 64.8332)
  point P92 (4.8693, 69)
  point P93 (4.7919, 67)
  dimension "d0" = 10
  dimension "d1" = 67
  dimension "d2" = 0
  dimension "d38" = 4
  dimension "d39" = 3
  dimension "d40" = 5
  dimension "d41" = 2
  dimension "d42" = 7
  dimension "d45" = 360
  constraints: 1056 end point, 45 midpoint, 44 point on line, 5 horizontal, 4 parallel, 3 perpendicular, 1057 other
  measures "d0" distance of L0.end L0.start
  measures "d1" distance from line of point (0, 0) L0
  measures "d2" horizontal distance of point (0, 0) L1.start
  measures "d38" distance of L1.end L2.end
  measures "d39" distance of L5.end L6.end
  measures "d40" distance from line of L1.start L2
  measures "d41" distance of L8.end L9.end
  measures "d42" distance from line of L5.end L11
extrude "Extrusion1" add sketch "Sketch1" along normal mid plane 12 contours L5 L10 L524 L516 L0 | L0 L12 L19 L18 L2 L4 L5 | L12 L17 L18 L2 L0 | L0 L2 L18 L19 L12 | L516 L524 L10 L11 L0 | L0 L11 L10 L524 L525 L526 L521 L516 | L521 L522 L512 L504 L516 | L12 L24 L31 L30 L20 L21 L22 L17 | L24 L29 L30 L20 L12 | L12 L20 L30 L31 L24 | L516 L523 L522 L512 L513 L514 L509 L504 | L504 L512 L522 L523 L516 | L509 L510 L500 L492 L504 | L24 L36 L43 L42 L32 L33 L34 L29 | L36 L41 L42 L32 L24 | L24 L32 L42 L43 L36 | L504 L511 L510 L500 L501 L502 L497 L492 | L492 L500 L510 L511 L504 | L497 L498 L488 L480 L492 | L36 L48 L55 L54 L44 L45 L46 L41 | L48 L53 L54 L44 L36 | L36 L44 L54 L55 L48 | L492 L499 L498 L488 L489 L490 L485 L480 | L480 L488 L498 L499 L492 | L485 L486 L476 L468 L480 | L48 L60 L67 L66 L56 L57 L58 L53 | L60 L65 L66 L56 L48 | L48 L56 L66 L67 L60 | L480 L487 L486 L476 L477 L478 L473 L468 | L468 L476 L486 L487 L480 | L473 L474 L464 L456 L468 | L60 L72 L79 L78 L68 L69 L70 L65 | L72 L77 L78 L68 L60 | L60 L68 L78 L79 L72 | L468 L475 L474 L464 L465 L466 L461 L456 | L456 L464 L474 L475 L468 | L461 L462 L452 L444 L456 | L72 L84 L91 L90 L80 L81 L82 L77 | L84 L89 L90 L80 L72 | L72 L80 L90 L91 L84 | L456 L463 L462 L452 L453 L454 L449 L444 | L444 L452 L462 L463 L456 | L449 L450 L440 L432 L444 | L84 L96 L103 L102 L92 L93 L94 L89 | L96 L101 L102 L92 L84 | L84 L92 L102 L103 L96 | L444 L451 L450 L440 L441 L442 L437 L432 | L432 L440 L450 L451 L444 | L437 L438 L428 L420 L432 | L96 L108 L115 L114 L104 L105 L106 L101 | L108 L113 L114 L104 L96 | L96 L104 L114 L115 L108 | L432 L439 L438 L428 L429 L430 L425 L420 | L420 L428 L438 L439 L432 | L425 L426 L416 L408 L420 | L108 L120 L127 L126 L116 L117 L118 L113 | L120 L125 L126 L116 L108 | L108 L116 L126 L127 L120 | L420 L427 L426 L416 L417 L418 L413 L408 | L408 L416 L426 L427 L420 | L413 L414 L404 L396 L408 | L120 L132 L139 L138 L128 L129 L130 L125 | L132 L137 L138 L128 L120 | L120 L128 L138 L139 L132 | L408 L415 L414 L404 L405 L406 L401 L396 | L396 L404 L414 L415 L408 | L401 L402 L392 L384 L396 | L132 L144 L151 L150 L140 L141 L142 L137 | L144 L149 L150 L140 L132 | L132 L140 L150 L151 L144 | L396 L403 L402 L392 L393 L394 L389 L384 | L384 L392 L402 L403 L396 | L389 L390 L380 L372 L384 | L144 L156 L163 L162 L152 L153 L154 L149 | L156 L161 L162 L152 L144 | L144 L152 L162 L163 L156 | L384 L391 L390 L380 L381 L382 L377 L372 | L372 L380 L390 L391 L384 | L377 L378 L368 L360 L372 | L156 L168 L175 L174 L164 L165 L166 L161 | L168 L173 L174 L164 L156 | L156 L164 L174 L175 L168 | L372 L379 L378 L368 L369 L370 L365 L360 | L360 L368 L378 L379 L372 | L365 L366 L356 L348 L360 | L168 L180 L187 L186 L176 L177 L178 L173 | L180 L185 L186 L176 L168 | L168 L176 L186 L187 L180 | L360 L367 L366 L356 L357 L358 L353 L348 | L348 L356 L366 L367 L360 | L353 L354 L344 L336 L348 | L180 L192 L199 L198 L188 L189 L190 L185 | L192 L197 L198 L188 L180 | L180 L188 L198 L199 L192 | L348 L355 L354 L344 L345 L346 L341 L336 | L336 L344 L354 L355 L348 | L341 L342 L332 L324 L336 | L192 L204 L211 L210 L200 L201 L202 L197 | L204 L209 L210 L200 L192 | L192 L200 L210 L211 L204 | L336 L343 L342 L332 L333 L334 L329 L324 | L324 L332 L342 L343 L336 | L329 L330 L320 L312 L324 | L204 L216 L223 L222 L212 L213 L214 L209 | L216 L221 L222 L212 L204 | L204 L212 L222 L223 L216 | L324 L331 L330 L320 L321 L322 L317 L312 | L312 L320 L330 L331 L324 | L317 L318 L308 L300 L312 | L216 L228 L235 L234 L224 L225 L226 L221 | L228 L233 L234 L224 L216 | L216 L224 L234 L235 L228 | L312 L319 L318 L308 L309 L310 L305 L300 | L300 L308 L318 L319 L312 | L305 L306 L296 L288 L300 | L228 L240 L247 L246 L236 L237 L238 L233 | L240 L245 L246 L236 L228 | L228 L236 L246 L247 L240 | L300 L307 L306 L296 L297 L298 L293 L288 | L288 L296 L306 L307 L300 | L293 L294 L284 L276 L288 | L240 L252 L259 L258 L248 L249 L250 L245 | L252 L257 L258 L248 L240 | L240 L248 L258 L259 L252 | L288 L295 L294 L284 L285 L286 L281 L276 | L276 L284 L294 L295 L288 | L281 L282 L272 L264 L276 | L252 L264 L271 L270 L260 L261 L262 L257 | L264 L269 L270 L260 L252 | L252 L260 L270 L271 L264 | L276 L283 L282 L272 L273 L274 L269 L264 | L264 L272 L282 L283 L276
sketch "Sketch4" plane through (-2, 69, 6) normal (0, 1, 0) x (1, 0, 0)
  line L0 (-0.8936, 5.8202) -> (-0.8936, 1.8202)
  line L1 (0, 8.2) -> (6.8693, 8.2)
  line L2 (6.8693, 8.2) -> (6.8693, 3.8)
  line L3 (6.8693, 3.8) -> (0, 3.8)
  line L4 (0, 3.8) -> (0, 8.2)
  line L5 (0, 12) -> (0, 0) projected
  line L6 (6.8693, 12) -> (6.8693, 0) projected
  point P0 (2, 6)
  dimension "d55" = 4.4
  dimension "d56" = 2.2
  dimension "d57" = 0
  dimension "d58" = 0
  constraints: 10 end point, 2 parallel, 1 horizontal, 1 perpendicular
  measures "d55" distance between parallel lines of L3 L1
  measures "d56" distance from line of point (2, 6) L1
  measures "d57" distance between parallel lines of L5 L4
  measures "d58" distance between parallel lines of L2 L6
extrude "Extrusion4" cut sketch "Sketch4" against normal blind 12
pattern_circular "Circular Pattern2" count 44 over 360 about axis through (0, 0, -10) along (0, 0, 1) of "Extrusion4"
body "Solid1"
